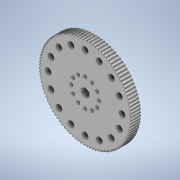
# Autodesk Inventor part: 100ToothBase
Saved by Autodesk Inventor 2020 (Build 240168000, 168)
## iProperties
Created: 2020-01-19
Part Number: 100ToothBase
Material: Generic
Document SubType Name: Modeling
Designer: srini
Density: 1 g/cm^3
Appearance: Default
Author: srini
Autodesk Inventor part; units mm, degrees
ref_plane "YZ Plane" through (0, 0, 0) normal (1, 0, 0) x (0, 1, 0)
ref_plane "XZ Plane" through (0, 0, 0) normal (0, 1, 0) x (-1, 0, 0)
ref_plane "XY Plane" through (0, 0, 0) normal (0, 0, 1) x (1, 0, 0)
sketch "Sketch1" plane through (0, 0, 0) normal (0, 0, 1) x (1, 0, 0)
  circle A0 centre (0, 0) radius 79.006
  dimension "d0" = 158.012
  constraints: 1 centre point, 1 coincident
  measures "d0" diameter of A0
extrude "Extrusion1" add sketch "Sketch1" along normal blind 16
sketch "Sketch2" plane through (0, 0, 16) normal (0, 0, 1) x (1, 0, 0)
  arc A0 (-1.543, 78.4662) -> (1.543, 78.4662) centre (0, 78.4662) ccw
  line L0 (-2.0693, 78.9789) -> (-2.0693, 80.609)
  line L1 (-2.0693, 80.609) -> (2.0693, 80.609)
  line L2 (2.0693, 80.609) -> (2.0693, 78.9789)
  circle A1 centre (0, 0) radius 79.006 construction
  arc A2 (-1.543, 78.4662) -> (-2.0693, 78.9789) centre (-2.0559, 78.4662) ccw
  arc A3 (2.0693, 78.9789) -> (1.543, 78.4662) centre (2.0559, 78.4662) ccw
  dimension "d3" = 1.543
  dimension "d47" = 2.0828
  constraints: 8 point on circle, 6 end point, 3 centre point, 3 tangent, 2 horizontal alignment, 2 vertical, 1 equal radius, 1 perpendicular, 1 vertical alignment
  measures "d3" radius of A0
extrude "Extrusion2" cut sketch "Sketch2" against normal through all
pattern_circular "Circular Pattern1" count 100 over 360 about axis through (0, 0, 0) along (0, 0, 1) of "Extrusion2"
sketch "Sketch7" plane through (0, 0, 16) normal (0, 0, 1) x (1, 0, 0)
  circle A0 centre (0, 63.4238) radius 4.8875
  circle A1 centre (-24.2712, 58.596) radius 4.8875
  circle A2 centre (-44.8474, 44.8474) radius 4.8875
  circle A3 centre (-58.596, 24.2712) radius 4.8875
  circle A4 centre (-63.4238, 0) radius 4.8875
  circle A5 centre (-58.596, -24.2712) radius 4.8875
  circle A6 centre (-44.8474, -44.8474) radius 4.8875
  circle A7 centre (-24.2712, -58.596) radius 4.8875
  circle A8 centre (0, -63.4238) radius 4.8875
  circle A9 centre (24.2712, -58.596) radius 4.8875
  circle A10 centre (44.8474, -44.8474) radius 4.8875
  circle A11 centre (58.596, -24.2712) radius 4.8875
  circle A12 centre (63.4238, 0) radius 4.8875
  circle A13 centre (58.596, 24.2712) radius 4.8875
  circle A14 centre (44.8474, 44.8474) radius 4.8875
  circle A15 centre (24.2712, 58.596) radius 4.8875
  point P0 (0, 0)
  dimension "d50" = 9.775
  dimension "d51" = 63.4238
  dimension "d54" = 360
  constraints: 16 centre point, 1 vertical alignment, 33 other
  measures "d50" diameter of A0
  measures "d51" distance of point (0, 0) A0.centre
extrude "Extrusion7" cut sketch "Sketch7" against normal through all
sketch "Sketch8" plane through (0, 0, 16) normal (0, 0, 1) x (1, 0, 0)
  circle A0 centre (0, 23.8125) radius 2.5781
  circle A1 centre (-11.9062, 20.6222) radius 2.5781
  circle A2 centre (-20.6222, 11.9063) radius 2.5781
  circle A3 centre (-23.8125, 0) radius 2.5781
  circle A4 centre (-20.6222, -11.9062) radius 2.5781
  circle A5 centre (-11.9063, -20.6222) radius 2.5781
  circle A6 centre (0, -23.8125) radius 2.5781
  circle A7 centre (11.9062, -20.6222) radius 2.5781
  circle A8 centre (20.6222, -11.9063) radius 2.5781
  circle A9 centre (23.8125, 0) radius 2.5781
  circle A10 centre (20.6222, 11.9062) radius 2.5781
  circle A11 centre (11.9063, 20.6222) radius 2.5781
  line L0 (-6.35, -3.6662) -> (-6.35, 3.6662)
  line L1 (-6.35, 3.6662) -> (0, 7.3323)
  line L2 (0, 7.3323) -> (6.35, 3.6662)
  line L3 (6.35, 3.6662) -> (6.35, -3.6662)
  line L4 (6.35, -3.6662) -> (0, -7.3323)
  line L5 (0, -7.3323) -> (-6.35, -3.6662)
  point P0 (0, 0)
  point P1 (0, 0)
  dimension "d58" = 5.1562
  dimension "d59" = 23.8125
  dimension "d62" = 360
  dimension "d64" = 12.7
  constraints: 12 centre point, 12 end point, 1 coincident, 1 vertical, 1 vertical alignment, 38 other
  measures "d58" diameter of A0
  measures "d59" distance of point (0, 0) A0.centre
  measures "d64" distance between parallel lines of L3 L0
extrude "Extrusion8" cut sketch "Sketch8" against normal through all
body "Solid1"
